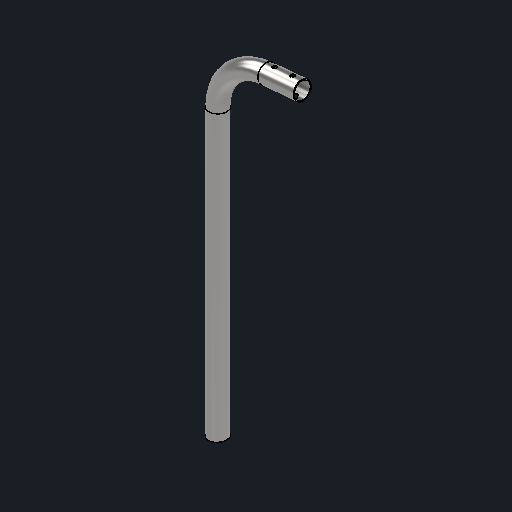
# Autodesk Inventor part: Leg
Saved by Autodesk Inventor 2026.2 (Build 302298000, 298)
## iProperties
Created: 2026-10-01
Part Number: Leg
Material: Steel, Carbon
Document SubType Name: Modeling
Designer: Joshua Eah
Density: 7.85 g/cm^3
Appearance: Semi-Polished
Mass: 420.09 g
Surface Area: 863.133 cm^2
Volume: 53.5147 cm^3
Author: Joshua Eah
Autodesk Inventor part; units mm, degrees
ref_plane "YZ Plane" through (0, 0, 0) normal (1, 0, 0) x (0, 1, 0)
ref_plane "XZ Plane" through (0, 0, 0) normal (0, 1, 0) x (-1, 0, 0)
sketch "Sketch1" plane through (0, 0, 0) normal (0, 1, 0) x (-1, 0, 0)
  circle A0 centre (0, 0) radius 12.7
  point P0 (12.7, 0)
  dimension "d1" = 25.4
  constraints: 2 horizontal alignment, 1 coincident, 2 other
sketch "Sketch2" plane through (0, 0, 0) normal (0, 0, 1) x (1, 0, 0)
  line L0 (0, 0) -> (0, 406.4)
  line L1 (0, 0) -> (406.4, 0) construction
  arc A0 (69.5587, 482.31) -> (0, 406.4) centre (76.2, 406.4) ccw
  line L2 (0, 406.4) -> (76.2, 406.4) construction
  line L3 (69.5587, 482.31) -> (76.2, 406.4) construction
  line L4 (69.5587, 482.31) -> (120.1654, 486.7375)
  dimension "d2" = 406.4
  dimension "d3" = 90
  dimension "d5" = 76.2
  dimension "d6" = 85
  dimension "d63" = 50.8
  constraints: 10 end point, 2 perpendicular, 2 point on circle, 1 centre point, 1 coincident, 1 horizontal, 1 tangent
  measures "d2" distance of L0.start L0.end
  measures "d3" angle of L1 L0
  measures "d5" radius of A0
  measures "d6" angle of L3 L2
  measures "d63" distance of L3.start L4.end
sweep "Sweep4" add profiles "Sketch1" path "Sketch2"
shell "Shell3" thickness 1.2446 removed faces 2 at (119.8785, 490.0167, 3.8203) at (0.5595, 0, -2.1641)
ref_plane "Work Plane7" through (-12.7, 0, 0) normal (0.0871557, -0.9961947, 0) x (0, 0, 1)
split "Split1" plane through (-12.7, 0, 0) removes the side toward (0.0871557, -0.9961947, 0)
ref_plane "Work Plane8" through (70.6656, 469.6584, 0) normal (0.0871557, -0.9961947, 0) x (0, 0, 1)
sketch "Sketch9" plane through (70.6656, 469.6584, 0) normal (0.0871557, -0.9961947, 0) x (0, 0, 1)
  line L0 (-12.7, -50.8) -> (12.7, -50.8) construction
  line L1 (-12.7, 0) -> (12.7, 0) construction
  line L2 (0, 0) -> (0, -50.8)
  point P0 (0, -12.7)
  point P1 (0, -25.4)
  dimension "d75" = 25.4
  constraints: 3 midpoint, 2 end point, 1 point on line
  measures "d75" diameter of point (0, -12.7) point (0, -25.4)
hole "Hole3" at (83.3173, 470.7652, 0) direction (-0.0871557, 0.9961947, 0) diameter 5.7912 end through all countersink diameter 11.1252 countersink angle 82
pattern_linear "Rectangular Pattern1" count 2 spacing 25.4 along (0.9961947, 0.0871557, 0) of "Hole3"
equation "\"d1\" = tubeOD"
equation "\"d6\" = bendAngle"
equation "\"d63\" = attachmentLength"
equation "\"d64\" = tubeT"
equation "\"tubeOD\" = 25.4"
equation "\"tubeT\" = 1.2446"
equation "\"attachmentLength\" = 50.8"
equation "\"bendAngle\" = 85deg"
body "Solid1"
body "Solid5"
